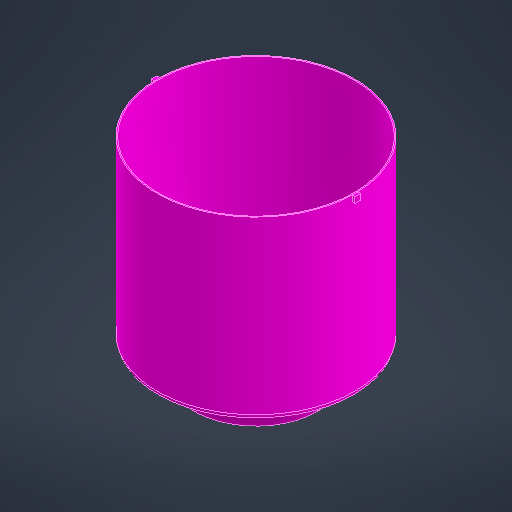
# Autodesk Inventor part: Zásobník oprava
Saved by Autodesk Inventor 2026.2 (Build 302298000, 298)
## iProperties
Created: 2025-10-01
Part Number: Zásobník oprava
Material: Všeobecné
Document SubType Name: Modeling
Designer: cerna
Density: 1 g/cm^3
Appearance: Purpurová
Author: cerna
Autodesk Inventor part; units mm, degrees
ref_plane "XZ Plane" through (0, 0, 0) normal (0, 1, 0) x (-1, 0, 0)
sketch "Náčrt10" plane through (0, 0, 0) normal (0, 1, 0) x (-1, 0, 0)
  circle A0 centre (0, 0) radius 52.5
  circle A1 centre (0, 0) radius 53
  line L0 (43, 24) -> (-29, 24)
  line L1 (-29, 24) -> (-29, -2)
  line L2 (-29, -2) -> (43, -2)
  line L3 (43, -2) -> (43, 24)
  line L4 (42, -1) -> (-28, -1)
  line L5 (-28, 23) -> (42, 23)
  line L6 (42, 23) -> (42, -1)
  line L7 (0, -74.2) -> (0, 74.2) projected
  line L8 (-74.2, 0) -> (74.2, 0) projected
  line L9 (-28, 23) -> (-28, -1)
  point P0 (-52.5, 0)
  point P1 (-53, 0)
  point P2 (0, -53)
  point P3 (0, -52.5)
  dimension "d54" = 105
  dimension "d55" = 106
  dimension "d56" = 72
  dimension "d57" = 26
  dimension "d58" = 1
  dimension "d59" = 1
  dimension "d95" = 28
  dimension "d96" = 1
  dimension "d97" = 1
  constraints: 16 end point, 4 parallel, 2 centre point, 2 coincident, 1 horizontal, 1 perpendicular, 1 other
  measures "d54" diameter of A0
  measures "d55" diameter of A1
  measures "d56" distance of L2.end L1.end
  measures "d57" distance of L1.end L0.end
  measures "d58" distance between parallel lines of L2 L4
  measures "d59" distance between parallel lines of L8 L4
  measures "d95" distance between parallel lines of L7 L9
  measures "d96" distance between parallel lines of L9 L1
  measures "d97" distance between parallel lines of L0 L5
extrude "Vysunutí12" add sketch "Náčrt10" along normal blind 2 contours L8 A1 L7 A0 | A0 L7 A1 L8 | A0 L8 A1 L7 | L7 A1 L8 A0 | L8 L6 L5 L7 L0 L3 | L3 L2 L7 L4 L6 L8 | L7 L5 L9 L8 L1 L0 | L2 L1 L8 L9 L4 L7
sketch "Náčrt12" plane through (0, 2, 0) normal (0, 1, 0) x (1, 0, 0)
  circle A0 centre (0, 0) radius 52.5
  circle A1 centre (0, 0) radius 53
  line L0 (29, -24) -> (29, 2) projected
  line L1 (-43, -24) -> (29, -24) projected
  line L2 (-43, 2) -> (-43, -24) projected
  line L3 (29, 2) -> (-43, 2) projected
  line L4 (-43, 2) -> (29, 2)
  line L5 (29, 2) -> (29, -24)
  line L6 (29, -24) -> (-43, -24)
  line L7 (-43, -24) -> (-43, 2)
  line L8 (-43, -24) -> (29, -24)
  line L9 (29, -24) -> (29, 2)
  line L10 (29, 2) -> (-43, 2)
  line L11 (-43, 2) -> (-43, -24)
  line L12 (-42, -23) -> (28, -23)
  line L13 (28, -23) -> (28, 1)
  line L14 (28, 1) -> (-42, 1)
  line L15 (-42, 1) -> (-42, -23)
  line L16 (-39.1162, 1) -> (-42, 1)
  line L17 (-43, 1) -> (-42, 1)
  line L18 (28, 1) -> (29, 1)
  line L19 (-43, -24) -> (29, -24)
  line L20 (29, -24) -> (29, 2)
  line L21 (29, 2) -> (-43, 2)
  line L22 (-43, 2) -> (-43, -24)
  point P0 (29, 1)
  dimension "d68" = 105
  dimension "d69" = 106
  dimension "d98" = 1
  constraints: 38 end point, 6 parallel, 4 perpendicular, 4 point on line, 3 horizontal, 2 centre point, 2 coincident, 1 collinear, 3 other
  measures "d68" diameter of A0
  measures "d69" diameter of A1
  measures "d98" distance between parallel lines of L2 L15
extrude "Vysunutí13" add sketch "Náčrt12" along normal blind 24 contours A1 | L1 L2 L17 L15 L12 L13 L18 L0
ref_plane "Pracovní rovina7" through (53, 0, 0) normal (1, 0, 0) x (0, 1, 0)
sketch "Náčrt13" plane through (53, 0, 0) normal (1, 0, 0) x (0, 1, 0)
  line L0 (26, -53) -> (26, 53) projected
  line L1 (0, -53) -> (0, 53) projected
  line L2 (-6, 0) -> (36, 0) projected
  line L3 (0, 74.2) -> (0, -74.2) projected
  line L4 (3, 2.45) -> (8, 2.45)
  line L5 (8, 2.45) -> (8, -2.45)
  line L6 (8, -2.45) -> (3, -2.45)
  line L7 (3, -2.45) -> (3, 2.45)
  point P0 (0, 0)
  dimension "d72" = 5
  dimension "d73" = 4.9
  dimension "d74" = 3
  constraints: 8 end point, 2 parallel, 1 horizontal, 1 perpendicular, 1 other
  measures "d72" distance of L5.end L6.end
  measures "d73" distance of L4.end L5.end
  measures "d74" distance between parallel lines of L7 L1
extrude "Vysunutí14" add sketch "Náčrt13" along normal blind 2.5
pattern_circular "Kruhové pole1" count 2 over 360 about axis through (0, -10, 0) along (0, 1, 0) of "Vysunutí14"
sketch "Náčrt14" plane through (0, 26, 0) normal (0, 1, 0) x (1, 0, 0)
  line L0 (-43, 2) -> (-43, 1) projected
  line L1 (29, 2) -> (-43, 2) projected
  line L2 (29, 1) -> (29, 2) projected
  circle A0 centre (0, 0) radius 85
  line L3 (-43, 1) -> (-43, -24) projected
  line L4 (-43, -24) -> (29, -24) projected
  line L5 (29, -24) -> (29, 1) projected
  line L6 (-36.5, 1) -> (36.5, 1)
  line L7 (28, -23) -> (-42, -23) projected
  line L8 (-42, -23) -> (-42, 1) projected
  line L9 (28, 1) -> (28, -23) projected
  line L10 (-42, 1) -> (28, 1) projected
  line L11 (28, 1) -> (29, 1) projected
  line L12 (-43, -24) -> (34, -24)
  line L13 (29, 2) -> (-46, 2)
  line L14 (-42, 1) -> (28, 1) projected
  line L15 (-42, -23) -> (28, -23)
  line L16 (28, -23) -> (28, 1)
  line L17 (-42, 1) -> (-42, -23)
  line L18 (-42, -23) -> (28, -23)
  line L19 (28, -23) -> (28, 1)
  line L20 (28, 1) -> (-42, 1)
  line L21 (-42, 1) -> (-42, -23)
  line L22 (-42, 1) -> (-43, 1) projected
  line L23 (29, 1) -> (28, 1) projected
  line L24 (-43, 1) -> (-42, 1) projected
  point P0 (-42, 1)
  point P1 (28, 1)
  point P2 (34.0001, 1)
  point P3 (28, 1)
  point P4 (28, 1)
  point P5 (35, 1)
  point P6 (-43, 1)
  dimension "d80" = 170
  constraints: 20 end point, 4 horizontal, 4 parallel, 2 perpendicular, 1 centre point
  measures "d80" diameter of A0
extrude "Vysunutí15" add sketch "Náčrt14" along normal blind 2 contours L1 L2 L6 L10 L22 L0 | L22 L8 L7 L9 L6 L5 L4 L3 | A0
sketch "Náčrt15" plane through (0, 28, 0) normal (0, 1, 0) x (1, 0, 0)
  circle A0 centre (0, 0) radius 85
  circle A1 centre (0, 0) radius 84
  dimension "d83" = 170
  dimension "d84" = 168
  constraints: 2 centre point, 2 coincident
  measures "d83" diameter of A0
  measures "d84" diameter of A1
extrude "Vysunutí16" add sketch "Náčrt15" along normal blind 150
fillet "Zaoblení7" radius 5 1 edges at (-85, 26, 0)
ref_plane "Pracovní rovina8" through (85, 26, 0) normal (1, 0, 0) x (0, 1, 0)
sketch "Náčrt16" plane through (85, 26, 0) normal (1, 0, 0) x (0, 1, 0)
  line L0 (152, 84) -> (152, -84) projected
  line L1 (152, 2.5) -> (147.1, 2.5)
  line L2 (147.1, 2.5) -> (147.1, -2.5)
  line L3 (147.1, -2.5) -> (152, -2.5)
  line L4 (152, -2.5) -> (152, 2.5)
  line L5 (-26, 119) -> (-26, -119) projected
  line L6 (-66.4, 0) -> (188.4, 0) projected
  point P0 (-26, 0)
  point P1 (152, -2.5)
  dimension "d88" = 4.9
  dimension "d89" = 5
  constraints: 8 end point, 2 parallel, 1 horizontal, 1 perpendicular, 1 point on line, 1 other
  measures "d88" distance of L3.end L2.end
  measures "d89" distance of L2.end L1.end
extrude "Vysunutí17" add sketch "Náčrt16" along normal blind 2.5
pattern_circular "Kruhové pole2" count 2 over 360 about axis through (0, -10, 0) along (0, 1, 0) of "Vysunutí17"
